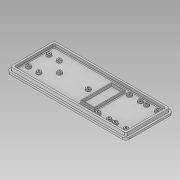
# Autodesk Inventor part: BASE INFERIOR
Saved by Autodesk Inventor 2019 (Build 230136000, 136)
## iProperties
Created: 2019-07-31
Part Number: BASE INFERIOR
Material: Genérico
Document SubType Name: Modeling
Designer: Luis Pujol
Density: 1 g/cm^3
Appearance: Valor por defecto
Author: Luis Pujol
## iProperties of the stored document BASE INFERIOR_3DPrint.ipt
Created: 2019-07-31
Part Number: BASE INFERIOR_3DPrint
Material: Genérico
Document SubType Name: Modeling
Designer: Luis Pujol
Density: 1 g/cm^3
Appearance: Valor por defecto
Author: Luis Pujol
Autodesk Inventor part; units mm, degrees
ref_plane "YZ Plane" through (0, 0, 0) normal (1, 0, 0) x (0, 1, 0)
ref_plane "XZ Plane" through (0, 0, 0) normal (0, 1, 0) x (-1, 0, 0)
ref_plane "XY Plane" through (0, 0, 0) normal (0, 0, 1) x (1, 0, 0)
sketch "Boceto1" plane through (0, 0, 0) normal (0, 1, 0) x (-1, 0, 0)
  line L0 (78, 22) -> (57, 22)
  line L1 (57, 22) -> (57, -22)
  line L2 (57, -22) -> (78, -22)
  line L3 (78, -22) -> (78, 22)
  line L4 (78, 22) -> (57, -22) construction
  line L5 (57, 22) -> (78, -22) construction
  line L6 (52, 18) -> (-5, 18)
  line L7 (-5, 18) -> (-5, -18)
  line L8 (-5, -18) -> (52, -18)
  line L9 (52, -18) -> (52, 18)
  line L10 (52, 18) -> (-5, -18) construction
  line L11 (-5, 18) -> (52, -18) construction
  line L12 (-10, 21.5) -> (-28, 21.5)
  line L13 (-28, 21.5) -> (-28, -21.5)
  line L14 (-28, -21.5) -> (-10, -21.5)
  line L15 (-10, -21.5) -> (-10, 21.5)
  line L16 (-10, 21.5) -> (-28, -21.5) construction
  line L17 (-28, 21.5) -> (-10, -21.5) construction
  line L18 (-33, 25) -> (-53, 25)
  line L19 (-53, 25) -> (-53, -25)
  line L20 (-53, -25) -> (-33, -25)
  line L21 (-33, -25) -> (-33, 25)
  line L22 (-33, 25) -> (-53, -25) construction
  line L23 (-53, 25) -> (-33, -25) construction
  line L24 (-58, 25) -> (-78, 25)
  line L25 (-78, 25) -> (-78, -25)
  line L26 (-78, -25) -> (-58, -25)
  line L27 (-58, -25) -> (-58, 25)
  line L28 (-58, 25) -> (-78, -25) construction
  line L29 (-78, 25) -> (-58, -25) construction
  line L30 (87.5, 35) -> (-87.5, 35)
  line L31 (-87.5, 35) -> (-87.5, -35)
  line L32 (-87.5, -35) -> (87.5, -35)
  line L33 (87.5, -35) -> (87.5, 35)
  line L34 (87.5, 35) -> (-87.5, -35) construction
  line L35 (-87.5, 35) -> (87.5, -35) construction
  point P0 (0, 0)
  point P1 (67.5, 0)
  point P2 (23.5, 0)
  point P3 (-19, 0)
  point P4 (-43, 0)
  point P5 (-68, 0)
  point P6 (67.5, 0)
  point P7 (0, 0)
  point P8 (23.5, 0)
  point P9 (0, 0)
  point P10 (-19, 0)
  point P11 (-43, 0)
  point P12 (-68, 0)
  dimension "d0" = 21
  dimension "d1" = 44
  dimension "d2" = 57
  dimension "d3" = 36
  dimension "d4" = 18
  dimension "d5" = 43
  dimension "d6" = 20
  dimension "d7" = 50
  dimension "d8" = 20
  dimension "d9" = 50
  dimension "d10" = 5
  dimension "d11" = 5
  dimension "d12" = 5
  dimension "d13" = 5
  dimension "d15" = 9.5
  dimension "d16" = 9.5
  dimension "d17" = 70
  dimension "d18" = 175
  constraints: 72 end point, 19 midpoint, 12 parallel, 6 horizontal, 6 perpendicular, 5 horizontal alignment
  measures "d0" distance of L2.end L1.end
  measures "d1" distance of L1.end L0.end
  measures "d2" distance of L8.end L7.end
  measures "d3" distance of L7.end L6.end
  measures "d4" distance of L14.end L13.end
  measures "d5" distance of L13.end L12.end
  measures "d6" distance of L20.end L19.end
  measures "d7" distance of L19.end L18.end
  measures "d8" distance of L26.end L25.end
  measures "d9" distance of L25.end L24.end
  measures "d10" distance between parallel lines of L1 L9
  measures "d11" distance between parallel lines of L15 L7
  measures "d12" distance between parallel lines of L21 L13
  measures "d13" distance between parallel lines of L27 L19
  measures "d15" distance between parallel lines of L33 L3
  measures "d16" distance between parallel lines of L25 L31
  measures "d17" distance between parallel lines of L30 L32
  measures "d18" distance between parallel lines of L31 L33
extrude "Extrusión1" add sketch "Boceto1" along normal blind 2.8 contours L3 L2 L1 L0 | L9 L8 L7 L6 | L15 L14 L13 L12 | L21 L20 L19 L18 | L27 L26 L25 L24 | L33 L32 L31 L30
sketch "Boceto2" plane through (0, 2.8, 0) normal (0, 1, 0) x (1, 0, 0)
  line L0 (-87.5, -35) -> (87.5, -35) projected
  line L1 (87.5, -35) -> (87.5, 35) projected
  line L2 (87.5, 35) -> (-87.5, 35) projected
  line L3 (-87.5, 35) -> (-87.5, -35) projected
  line L4 (35, -23) -> (51, -23) construction
  line L5 (51, -23) -> (51, 23) construction
  line L6 (51, 23) -> (35, 23) construction
  line L7 (35, 23) -> (35, -23) construction
  line L8 (35, -23) -> (51, 23) construction
  line L9 (51, -23) -> (35, 23) construction
  line L10 (60, -23) -> (76, -23) construction
  line L11 (76, -23) -> (76, 23) construction
  line L12 (76, 23) -> (60, 23) construction
  line L13 (60, 23) -> (60, -23) construction
  line L14 (60, -23) -> (76, 23) construction
  line L15 (76, -23) -> (60, 23) construction
  line L16 (-2.5, -1.2609) -> (-2.5, 1.2609) construction
  line L17 (-44.5, 1.2609) -> (-44.5, -1.2609) construction
  line L18 (-75, -15) -> (-60, -15) construction
  line L19 (-60, -15) -> (-60, 15) construction
  line L20 (-60, 15) -> (-75, 15) construction
  line L21 (-75, 15) -> (-75, -15) construction
  line L22 (-75, -15) -> (-60, 15) construction
  line L23 (-60, -15) -> (-75, 15) construction
  circle A0 centre (-75, 15) radius 3
  circle A1 centre (-60, 15) radius 3
  circle A2 centre (-75, -15) radius 3
  circle A3 centre (-60, -15) radius 3
  circle A4 centre (-44.5, 0) radius 3
  circle A5 centre (-2.5, 0) radius 3
  circle A6 centre (35, 23) radius 3
  circle A7 centre (51, 23) radius 3
  circle A8 centre (35, -23) radius 3
  circle A9 centre (51, -23) radius 3
  circle A10 centre (60, -23) radius 3
  circle A11 centre (60, 23) radius 3
  circle A12 centre (76, 23) radius 3
  circle A13 centre (76, -23) radius 3
  point P0 (0, 0)
  point P1 (43, 0)
  point P2 (68, 0)
  point P3 (-67.5, 0)
  dimension "d21" = 16
  dimension "d22" = 46
  dimension "d23" = 16
  dimension "d24" = 46
  dimension "d25" = 42
  dimension "d26" = 15
  dimension "d27" = 30
  dimension "d28" = 6
  dimension "d29" = 6
  dimension "d30" = 6
  dimension "d31" = 6
  dimension "d32" = 6
  dimension "d33" = 6
  dimension "d34" = 6
  dimension "d35" = 6
  dimension "d36" = 6
  dimension "d37" = 6
  dimension "d38" = 6
  dimension "d39" = 6
  dimension "d40" = 6
  dimension "d41" = 6
  constraints: 40 end point, 14 centre point, 14 coincident, 8 midpoint, 7 parallel, 3 horizontal, 3 perpendicular
  measures "d21" distance of L6.end L5.end
  measures "d22" distance of L5.end L4.end
  measures "d23" distance of L12.end L11.end
  measures "d24" distance of L11.end L10.end
  measures "d25" distance of L17.start L16.end
  measures "d26" distance of L20.end L19.end
  measures "d27" distance of L19.end L18.end
  measures "d28" diameter of A0
  measures "d29" diameter of A1
  measures "d30" diameter of A2
  measures "d31" diameter of A3
  measures "d32" diameter of A4
  measures "d33" diameter of A5
  measures "d34" diameter of A6
  measures "d35" diameter of A7
  measures "d36" diameter of A8
  measures "d37" diameter of A9
  measures "d38" diameter of A10
  measures "d39" diameter of A11
  measures "d40" diameter of A12
  measures "d41" diameter of A13
extrude "Extrusión2" add sketch "Boceto2" along normal blind 2.8 contours A0 | A1 | A2 | A3 | A4 | A5 | A6 | A7 | A8 | A9 | A10 | A11 | A12 | A13
fillet "Empalme1" radius 0.5 28 edges at (-78, 5.6, 15) (-63, 5.6, 15) (-78, 5.6, -15) (-63, 5.6, -15) (-47.5, 5.6, 0) (-63, 2.8, -15) (-78, 2.8, -15) (-63, 2.8, 15) (-78, 2.8, 15) (-47.5, 2.8, 0) (-5.5, 5.6, 0) (-5.5, 2.8, 0) (32, 5.6, 23) (32, 2.8, 23) (48, 5.6, 23) (48, 2.8, 23) (57, 5.6, 23) (57, 2.8, 23) (73, 5.6, 23) (73, 2.8, 23) (48, 5.6, -23) (48, 2.8, -23) (57, 5.6, -23) (57, 2.8, -23) (73, 5.6, -23) (73, 2.8, -23) (32, 5.6, -23) (32, 2.8, -23)
fillet "Empalme2" radius 5 4 edges at (87.5, 1.4, 35) (87.5, 1.4, -35) (-87.5, 1.4, 35) (-87.5, 1.4, -35)
sketch "Boceto4" plane through (0, 2.8, 0) normal (0, 1, 0) x (1, 0, 0)
  circle A0 centre (76, 23) radius 3.5 projected
  circle A1 centre (51, 23) radius 3.5 projected
  circle A2 centre (60, -23) radius 3.5 projected
  circle A3 centre (35, -23) radius 3.5 projected
  circle A4 centre (-44.5, 0) radius 3.5 projected
  circle A5 centre (-60, -15) radius 3.5 projected
  circle A6 centre (-60, 15) radius 3.5 projected
  arc A7 (-82.5, 35) -> (-87.5, 30) centre (-82.5, 30) ccw projected
  line L0 (-87.5, 30) -> (-87.5, -30) projected
  arc A8 (-87.5, -30) -> (-82.5, -35) centre (-82.5, -30) ccw projected
  line L1 (-82.5, -35) -> (82.5, -35) projected
  arc A9 (82.5, -35) -> (87.5, -30) centre (82.5, -30) ccw projected
  line L2 (87.5, -30) -> (87.5, 30) projected
  arc A10 (87.5, 30) -> (82.5, 35) centre (82.5, 30) ccw projected
  line L3 (82.5, 35) -> (-82.5, 35) projected
  circle A11 centre (-75, 15) radius 3.5 projected
  circle A12 centre (-75, -15) radius 3.5 projected
  circle A13 centre (-2.5, 0) radius 3.5 projected
  circle A14 centre (51, -23) radius 3.5 projected
  circle A15 centre (76, -23) radius 3.5 projected
  circle A16 centre (60, 23) radius 3.5 projected
  circle A17 centre (35, 23) radius 3.5 projected
  arc A18 (-82.5, 32.18) -> (-84.68, 30) centre (-82.5, 30) ccw
  line L4 (-82.5, 32.18) -> (82.5, 32.18)
  arc A19 (84.68, 30) -> (82.5, 32.18) centre (82.5, 30) ccw
  line L5 (84.68, 30) -> (84.68, -30)
  arc A20 (82.5, -32.18) -> (84.68, -30) centre (82.5, -30) ccw
  line L6 (82.5, -32.18) -> (-82.5, -32.18)
  arc A21 (-84.68, -30) -> (-82.5, -32.18) centre (-82.5, -30) ccw
  line L7 (-84.68, -30) -> (-84.68, 30)
  line L8 (79.88, 29.38) -> (-79.88, 29.38)
  line L9 (-81.88, 27.38) -> (-81.88, -27.38)
  line L10 (-79.88, -29.38) -> (79.88, -29.38)
  line L11 (81.88, -27.38) -> (81.88, 27.38)
  arc A22 (-79.88, 29.38) -> (-81.88, 27.38) centre (-79.88, 27.38) ccw
  arc A23 (-81.88, -27.38) -> (-79.88, -29.38) centre (-79.88, -27.38) ccw
  arc A24 (79.88, -29.38) -> (81.88, -27.38) centre (79.88, -27.38) ccw
  arc A25 (81.88, 27.38) -> (79.88, 29.38) centre (79.88, 27.38) ccw
  point P0 (0, 0)
  dimension "d46" = 2.82
  dimension "d47" = 2.8
  dimension "d48" = 2
  constraints: 16 end point, 16 point on circle, 8 centre point, 8 tangent, 3 equal radius, 10 other
  measures "d46" radial gap between concentric circles of A7 A18
  measures "d47" distance between parallel lines of L4 L8
  measures "d48" radius of A22
extrude "Extrusión3" add sketch "Boceto4" along normal blind 5 contours L4 A19 L5 A20 L6 A21 L7 A18
sketch "Boceto5" plane through (0, 2.8, 0) normal (0, 1, 0) x (1, 0, 0)
  arc A0 (81.88, 27.38) -> (79.88, 29.38) centre (79.88, 27.38) ccw projected
  line L0 (79.88, 29.38) -> (-79.88, 29.38) projected
  arc A1 (-79.88, 29.38) -> (-81.88, 27.38) centre (-79.88, 27.38) ccw projected
  line L1 (-81.88, 27.38) -> (-81.88, -27.38) projected
  arc A2 (-81.88, -27.38) -> (-79.88, -29.38) centre (-79.88, -27.38) ccw projected
  line L2 (-79.88, -29.38) -> (79.88, -29.38) projected
  arc A3 (79.88, -29.38) -> (81.88, -27.38) centre (79.88, -27.38) ccw projected
  line L3 (81.88, -27.38) -> (81.88, 27.38) projected
  circle A4 centre (76, 23) radius 3.5 projected
  circle A5 centre (51, 23) radius 3.5 projected
  circle A6 centre (60, -23) radius 3.5 projected
  circle A7 centre (35, -23) radius 3.5 projected
  circle A8 centre (-44.5, 0) radius 3.5 projected
  circle A9 centre (-60, -15) radius 3.5 projected
  circle A10 centre (-60, 15) radius 3.5 projected
  circle A11 centre (-75, 15) radius 3.5 projected
  circle A12 centre (-75, -15) radius 3.5 projected
  circle A13 centre (-2.5, 0) radius 3.5 projected
  circle A14 centre (51, -23) radius 3.5 projected
  circle A15 centre (76, -23) radius 3.5 projected
  circle A16 centre (60, 23) radius 3.5 projected
  circle A17 centre (35, 23) radius 3.5 projected
  line L4 (10.2, -21.55) -> (27.8, -21.55)
  line L5 (27.8, -21.55) -> (27.8, 21.55)
  line L6 (27.8, 21.55) -> (10.2, 21.55)
  line L7 (10.2, 21.55) -> (10.2, -21.55)
  line L8 (10.2, -21.55) -> (27.8, 21.55) construction
  line L9 (27.8, -21.55) -> (10.2, 21.55) construction
  line L10 (29, -22.5) -> (9, -22.5)
  line L11 (9, -22.5) -> (9, 22.5)
  line L12 (9, 22.5) -> (29, 22.5)
  line L13 (29, 22.5) -> (29, -22.5)
  line L14 (29, -22.5) -> (9, 22.5) construction
  line L15 (9, -22.5) -> (29, 22.5) construction
  point P0 (0, 0)
  point P1 (19, 0)
  point P2 (19, 0)
  dimension "d51" = 17.6
  dimension "d52" = 43.1
  dimension "d53" = 20
  dimension "d54" = 45
  constraints: 24 end point, 6 midpoint, 4 parallel, 2 horizontal, 2 perpendicular
  measures "d51" distance of L6.end L5.end
  measures "d52" distance of L5.end L4.end
  measures "d53" distance of L11.end L12.end
  measures "d54" distance of L10.end L11.end
extrude "Extrusión4" add sketch "Boceto5" along normal blind 4 contours L10 L11 L12 L13
fillet "Empalme3" radius 1 4 edges at (29, 2.8, 0) (19, 2.8, 22.5) (9, 2.8, 0) (19, 2.8, -22.5)
fillet "Empalme4" radius 1 8 edges at (-81.2942, 2.8, -28.7942) (-81.88, 2.8, 0) (-81.2942, 2.8, 28.7942) (0, 2.8, 29.38) (81.2942, 2.8, 28.7942) (81.88, 2.8, 0) (81.2942, 2.8, -28.7942) (0, 2.8, -29.38)
sketch "Boceto6" plane through (-75, 5.6, -15) normal (0, 1, 0) x (1, 0, 0)
  circle A0 centre (0, 0) radius 2.5 projected
  circle A1 centre (15, 0) radius 2.5 projected
  circle A2 centre (30.5, -15) radius 2.5 projected
  circle A3 centre (15, -30) radius 2.5 projected
  circle A4 centre (0, -30) radius 2.5 projected
  circle A5 centre (72.5, -15) radius 2.5 projected
  circle A6 centre (110, 8) radius 2.5 projected
  circle A7 centre (126, 8) radius 2.5 projected
  circle A8 centre (135, 8) radius 2.5 projected
  circle A9 centre (151, 8) radius 2.5 projected
  circle A10 centre (110, -38) radius 2.5 projected
  circle A11 centre (126, -38) radius 2.5 projected
  circle A12 centre (135, -38) radius 2.5 projected
  circle A13 centre (151, -38) radius 2.5 projected
  point P0 (75, -15)
hole "Agujero1" at (-75, 5.6, -15) at (-60, 5.6, -15) at (-44.5, 5.6, 0) at (-60, 5.6, 15) at (-75, 5.6, 15) at (-2.5, 5.6, 0) at (35, 5.6, -23) at (51, 5.6, -23) at (60, 5.6, -23) at (76, 5.6, -23) at (35, 5.6, 23) at (51, 5.6, 23) at (60, 5.6, 23) at (76, 5.6, 23) direction (0, -1, 0) diameter 1.8 depth 5 tip angle 118 countersink diameter 2.5 countersink angle 90
